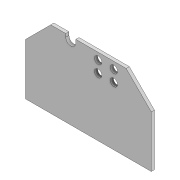
# Autodesk Inventor part: PSM_ECover
Saved by Autodesk Inventor 2022 (Build 260153000, 153)
## iProperties
Created: 2022-12-21
Part Number: PSM_ECover
Material: Generisch
Document SubType Name: Modeling
Designer: alexw
Density: 1 g/cm^3
Appearance: Vorgabe
Author: alexw
Autodesk Inventor part; units mm, degrees
ref_plane "YZ Plane" through (0, 0, 0) normal (1, 0, 0) x (0, 1, 0)
ref_plane "XZ Plane" through (0, 0, 0) normal (0, 1, 0) x (-1, 0, 0)
ref_plane "XY Plane" through (0, 0, 0) normal (0, 0, 1) x (1, 0, 0)
sketch "Skizze1" plane through (0, 0, 0) normal (0, 0, 1) x (1, 0, 0)
  line L0 (-100, 61) -> (100, 61)
  line L1 (100, 61) -> (100, -61)
  line L2 (100, -61) -> (-100, -61)
  line L3 (-100, -61) -> (-100, 61)
  line L4 (-100, 61) -> (100, -61) construction
  line L5 (100, 61) -> (-100, -61) construction
  line L6 (-100, 21) -> (-60, 61)
  line L7 (60, 61) -> (100, 21)
  circle A0 centre (15.5, 50) radius 5.9
  circle A1 centre (15.5, 32) radius 5.9
  circle A2 centre (40.5, 50) radius 5.9
  circle A3 centre (40.5, 32) radius 5.9
  line L8 (15.5, 50) -> (15.5, 32) construction
  line L9 (15.5, 50) -> (40.5, 50) construction
  line L10 (40.5, 50) -> (40.5, 32) construction
  line L11 (40.5, 32) -> (15.5, 32) construction
  line L12 (28, 50) -> (28, 32) construction
  line L13 (0, 61) -> (0, -61) construction
  line L14 (15.5, 41) -> (40.5, 41) construction
  arc A4 (-36, 56) -> (-20, 56) centre (-28, 56) ccw
  line L15 (-36, 56) -> (-36, 61)
  line L16 (-20, 56) -> (-20, 61)
  point P0 (0, 0)
  dimension "d0" = 45
  dimension "d1" = 40
  dimension "d2" = 122
  dimension "d3" = 200
  dimension "d4" = 40
  dimension "d5" = 45
  dimension "d8" = 11.8
  dimension "d9" = 11.8
  dimension "d10" = 11.8
  dimension "d11" = 11.8
  dimension "d12" = 25
  dimension "d13" = 18
  dimension "d14" = 28
  dimension "d15" = 20
  dimension "d16" = 8
  dimension "d17" = 5
  dimension "d18" = 28
  constraints: 34 end point, 8 midpoint, 6 point on line, 5 centre point, 4 perpendicular, 3 parallel, 2 horizontal, 2 point on circle, 2 tangent, 1 vertical
  measures "d0" angle of L3 L6
  measures "d1" distance from line of L6.end L3
  measures "d2" distance of L2.end L0.start
  measures "d3" distance of L1.end L2.end
  measures "d4" distance of L0.end L7.start
  measures "d5" angle of L1 L7
  measures "d8" diameter of A0
  measures "d9" diameter of A1
  measures "d10" diameter of A2
  measures "d11" diameter of A3
  measures "d12" distance of L8.start L9.end
  measures "d13" distance of L8.start L8.end
  measures "d14" distance between parallel lines of L13 L12
  measures "d15" distance between parallel lines of L0 L14
  measures "d16" radius of A4
  measures "d17" distance from line of L0 A4.centre
  measures "d18" distance from line of L13 A4.centre
extrude "Extrusion1" add sketch "Skizze1" along normal blind 5 contours L0 L15 A4 L16 L7 L1 L2 L3 L6
equation "\"d18\" = d14"
